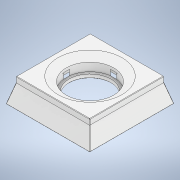
# Autodesk Inventor part: Cuerpo Lampara
Saved by Autodesk Inventor 2020.5 (Build 245400000, 400)
## iProperties
Created: 2019-10-08
Part Number: Cuerpo Lampara
Material: Generic
Document SubType Name: Modeling
Designer: aivel
Density: 1 g/cm^3
Appearance: Default
Sending System: SolidWorks 2017
Last Author: aleka
Last Saved: 2020-03-05
Author: aivel
Autodesk Inventor part; units mm, degrees
ref_plane "YZ Plane" through (0, 0, 0) normal (1, 0, 0) x (0, 1, 0)
ref_plane "XZ Plane" through (0, 0, 0) normal (0, 1, 0) x (-1, 0, 0)
ref_plane "Work Plane1" through (237.4877, 65, 162.655) normal (0, 1, 0) x (1, 0, 0)
sketch "Sketch1" plane through (237.4877, 65, 162.655) normal (0, 1, 0) x (1, 0, 0)
  line L0 (29.4023, 5.765) -> (28.4023, 5.765) construction
  line L1 (29.4023, 5.765) -> (5.6223, 29.545) construction
  line L2 (6.6223, 5.765) -> (5.6223, 5.765) construction
  line L3 (5.6223, 5.765) -> (29.4023, 29.545) construction
  circle A0 centre (17.5123, 17.655) radius 12.65
  line L4 (4.7623, 30.405) -> (30.2623, 30.405)
  line L5 (30.2623, 30.405) -> (30.2623, 4.905)
  line L6 (30.2623, 4.905) -> (4.7623, 4.905)
  line L7 (4.7623, 4.905) -> (4.7623, 30.405)
  line L8 (4.7623, 30.405) -> (30.2623, 30.405) construction
  line L9 (5.6223, 30.405) -> (5.6223, 27.405) construction
  line L10 (4.7623, 29.545) -> (7.7623, 29.545) construction
  line L11 (4.7623, 27.405) -> (7.7623, 30.405)
  line L12 (29.4023, 30.405) -> (29.4023, 27.405) construction
  line L13 (30.2623, 29.545) -> (27.2623, 29.545) construction
  line L14 (29.4023, 4.905) -> (29.4023, 7.905) construction
  line L15 (30.2623, 5.765) -> (27.2623, 5.765) construction
  line L16 (4.7623, 5.765) -> (7.7623, 5.765) construction
  line L17 (5.6223, 4.905) -> (5.6223, 7.905) construction
  line L18 (27.2623, 30.405) -> (30.2623, 27.405)
  line L19 (27.2623, 4.905) -> (30.2623, 7.905)
  line L20 (4.7623, 7.905) -> (7.7623, 4.905)
  line L21 (-0.1502, 35.4675) -> (35.1748, 35.4675)
  line L22 (35.1748, 35.4675) -> (35.1748, -0.1575)
  line L23 (35.1748, -0.1575) -> (-0.1502, -0.1575)
  line L24 (-0.1502, -0.1575) -> (-0.1502, 35.4675)
  line L25 (-0.1502, 35.4675) -> (35.1748, 35.4675) construction
  line L26 (-2.4877, 37.805) -> (37.5123, 37.805)
  line L27 (37.5123, 37.805) -> (37.5123, -2.495)
  line L28 (37.5123, -2.495) -> (-2.4877, -2.495)
  line L29 (-2.4877, -2.495) -> (-2.4877, 37.805)
  line L30 (-2.4877, 37.805) -> (37.5123, 37.805) construction
  line L31 (-2.4877, 37.805) -> (-0.1502, 35.4675)
  line L32 (37.5123, 37.805) -> (35.1748, 35.4675)
  line L33 (-0.1502, -0.1575) -> (-2.4877, -2.495)
  line L34 (35.1748, -0.1575) -> (37.5123, -2.495)
  circle A1 centre (17.5123, 17.655) radius 11.35
  line L35 (-37.4877, -37.345) -> (72.5123, -37.345)
  line L36 (72.5123, -37.345) -> (72.5123, 72.655)
  line L37 (72.5123, 72.655) -> (-37.4877, 72.655)
  line L38 (-37.4877, 72.655) -> (-37.4877, -37.345)
  line L39 (68.5123, 18.4852) -> (72.5123, 18.4852) projected
  line L40 (-37.4877, -37.345) -> (72.5123, -37.345) construction
  point P0 (35.1748, 35.4675)
  point P1 (37.5123, 37.805)
  point P2 (27.2623, 30.405)
  point P3 (7.7623, 30.405)
  point P4 (35.1748, 35.4675)
  point P5 (37.5123, 37.805)
  dimension "d48" = 110
  dimension "d50" = 110
  constraints: 76 end point, 16 point on line, 10 parallel, 9 perpendicular, 8 horizontal, 4 collinear, 2 centre point, 2 coincident, 1 midpoint, 1 vertical
  measures "d48" distance of L35.start L35.end
  measures "d50" distance of L36.end L35.end
extrude "Extrusion1" add sketch "Sketch1" against normal blind 6 contours L4 L18 L5 L19 L6 L20 L7 L11
extrude "Extrusion2" add sketch "Sketch1" along normal blind 2 from surface at -6 contours A0
sketch3d "3D Sketch7"
  line L0 (237.4877, 65, 162.655) -> (221, 5, 179.055)
sweep "Sweep7" add profiles "Sketch1" path "3D Sketch7" contours L23 L34 L28 L33
sketch3d "3D Sketch8"
  line L0 (272.5123, 65, 162.655) -> (289, 5, 179.055)
sweep "Sweep8" add profiles "Sketch1" path "3D Sketch8" contours L23 L34 L28 L33
sketch3d "3D Sketch9"
  line L0 (272.5123, 65, 162.655) -> (289, 5, 179.055)
sweep "Sweep9" add profiles "Sketch1" path "3D Sketch9" contours L32 L27 L34 L22
sketch3d "3D Sketch10"
  line L0 (272.5123, 65, 127.345) -> (289, 5, 110.945)
sweep "Sweep10" add profiles "Sketch1" path "3D Sketch10" contours L32 L27 L34 L22
sketch3d "3D Sketch11"
  line L0 (272.5123, 65, 127.345) -> (289, 5, 110.945)
sweep "Sweep11" add profiles "Sketch1" path "3D Sketch11" contours L31 L26 L32 L21
sketch3d "3D Sketch12"
  line L0 (237.4877, 65, 127.345) -> (221, 5, 110.945)
sweep "Sweep12" add profiles "Sketch1" path "3D Sketch12" contours L31 L26 L32 L21
sketch3d "3D Sketch13"
  line L0 (237.4877, 65, 127.345) -> (221, 5, 110.945)
sweep "Sweep13" add profiles "Sketch1" path "3D Sketch13" contours L24 L33 L29 L31
sketch3d "3D Sketch14"
  line L0 (237.4877, 65, 162.655) -> (221, 5, 179.055)
sweep "Sweep14" add profiles "Sketch1" path "3D Sketch14" contours L24 L33 L29 L31
extrude "Extrusion4" add sketch "Sketch1" along normal blind 3 contours L4 L11 L7 | L4 L18 L5 L19 L6 L20 L7 L11 | L4 L5 L18 | L20 L6 L7 | L5 L6 L19 | L31 L26 L32 L21 | L21 L22 L23 L24 | L24 L33 L29 L31 | L32 L27 L34 L22 | L23 L34 L28 L33
extrude "Extrusion5" cut sketch "Sketch1" along normal blind 50 from surface at -60 contours A0 | L4 L11 L7 | L4 L18 L5 L19 L6 L20 L7 L11 | L4 L5 L18 | L20 L6 L7 | L5 L6 L19 | L31 L26 L32 L21 | L21 L22 L23 L24 | L24 L33 L29 L31 | L32 L27 L34 L22 | L23 L34 L28 L33 | A1 | L38 L37 L36 L35
chamfer "Chamfer1" distance 0.25 angle 45 29 edges at (233.626, 60, 166.5167) (276.374, 60, 166.5167) (276.374, 60, 123.4833) (233.626, 60, 123.4833) (235, 66.5, 124.85) (275, 66.5, 124.85) (235, 66.5, 165.15) (275, 66.5, 165.15) (255, 68, 165.15) (275, 68, 145) (255, 68, 124.85) (235, 68, 145) (277.748, 55, 145) (255, 55, 167.8833) (232.252, 55, 145) (275.4105, 55, 145) (255, 55, 165.5458) (234.5895, 55, 145) (255, 55, 124.4542) (255, 55, 122.1167) (243.65, 59, 145) (243.75, 59, 133.75) (242.25, 59, 145) (243.75, 59, 156.25) (255, 59, 157.75) (266.25, 59, 156.25) (267.75, 59, 145) (266.25, 59, 133.75) (255, 59, 132.25)
extrude "Extrusion6" add sketch "Sketch1" against normal blind 1 contours L4 L11 L7 | L4 L5 L18 | L20 L6 L7 | L5 L6 L19 | L21 L22 L23 L24
sketch "Sketch2" plane through (255, 61, 145) normal (0, 1, 0) x (1, 0, 0)
  circle A0 centre (0, 0) radius 12.85
  point P0 (-255, 145)
  dimension "d100" = 25.7
  constraints: 1 centre point
  measures "d100" diameter of A0
extrude "Extrusion7" cut sketch "Sketch2" along normal blind 10
chamfer "Chamfer4" distance 4.5 distance2 2.5 1 edges at (242.15, 68, 145) measured on face at (241.65, 68, 145)
body "Solid1"
